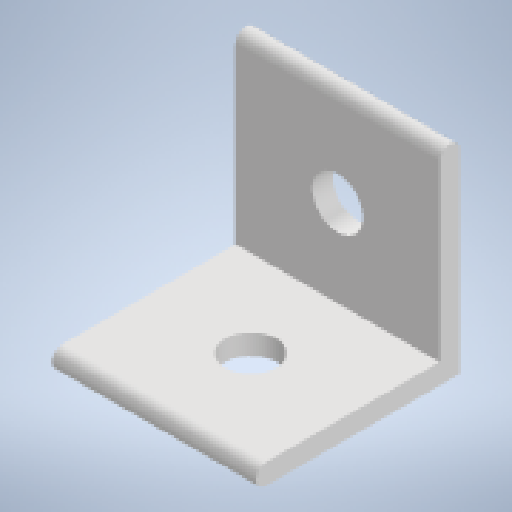
# Autodesk Inventor part: LVas
Saved by Autodesk Inventor 2025.2 (Build 292293000, 293)
## iProperties
Created: 2025-09-30
Part Number: LVas
Material: Generic
Document SubType Name: Modeling
Designer: MB
Density: 1 g/cm^3
Appearance: Default
Author: MB
Autodesk Inventor part; units mm, degrees
ref_plane "YZ Plane" through (0, 0, 0) normal (1, 0, 0) x (0, 1, 0)
ref_plane "XZ Plane" through (0, 0, 0) normal (0, 1, 0) x (-1, 0, 0)
ref_plane "XY Plane" through (0, 0, 0) normal (0, 0, 1) x (1, 0, 0)
sketch "Sketch1" plane through (0, 0, 0) normal (1, 0, 0) x (0, 1, 0)
  line L0 (0, -2) -> (0, -40)
  line L1 (0, -40) -> (38, -40)
  line L2 (4, -2) -> (4, -36)
  line L3 (4, -36) -> (38, -36)
  line L4 (2, 0) -> (2, 0)
  line L5 (40, -38) -> (40, -38)
  arc A0 (40, -38) -> (38, -36) centre (38, -38) ccw
  arc A1 (38, -40) -> (40, -38) centre (38, -38) ccw
  arc A2 (4, -2) -> (2, 0) centre (2, -2) ccw
  arc A3 (2, 0) -> (0, -2) centre (2, -2) ccw
  point P0 (0, 0)
  point P1 (40, -40)
  point P2 (2, 0)
  dimension "d0" = 40
  dimension "d1" = 40
  dimension "d2" = 4
  dimension "d3" = 2
  constraints: 12 end point, 8 point on circle, 8 tangent, 4 centre point, 4 point on line, 3 equal radius, 3 perpendicular, 1 horizontal, 1 vertical, 1 other
  measures "d0" distance of point (0, 0) L0.end
  measures "d1" distance of L0.end point (40, -40)
  measures "d2" distance between parallel lines of L0 L2
  measures "d3" radius of A0
extrude "Extrusion1" add sketch "Sketch1" along normal blind 40
sketch "Sketch2" plane through (0, 4, -2) normal (0, 1, 0) x (1, 0, 0)
  line L0 (0, 34) -> (0, 0) projected
  line L1 (0, 0) -> (40, 0) projected
  line L2 (40, 34) -> (40, 0) projected
  line L3 (0, 34) -> (40, 34) projected
  point P0 (0, -2)
  point P1 (20, 17)
hole "Hole1" at (20, 4, -19) direction (0, -1, 0) diameter 10 end through all
sketch "Sketch3" plane through (0, 4, -36) normal (0, 0, 1) x (1, 0, 0)
  line L0 (0, 34) -> (0, 0) construction
  line L1 (0, 0) -> (40, 0) construction
  line L2 (40, 34) -> (40, 0) construction
  line L3 (0, 34) -> (40, 34) construction
  point P0 (0, -4)
  point P1 (20, 17)
hole "Hole2" at (20, 21, -36) direction (0, 0, -1) diameter 10 end through all
body "Solid1"
